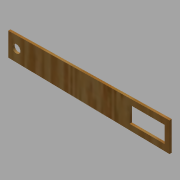
# Autodesk Inventor part: segment2b
Saved by Autodesk Inventor 2013 (Build 170138000, 138)
## iProperties
Created: 2014-10-09
Part Number: segment2b
Material: Plywood, Finish
Document SubType Name: Modeling
Designer: Masta
Density: 0.552 g/cm^3
Mass: 32.6528 g
Surface Area: 247.953 cm^2
Volume: 59.1536 cm^3
Author: Masta
Autodesk Inventor part; units mm, degrees
ref_plane "YZ Plane" through (0, 0, 0) normal (1, 0, 0) x (0, 1, 0)
ref_plane "XZ Plane" through (0, 0, 0) normal (0, 1, 0) x (-1, 0, 0)
ref_plane "XY Plane" through (0, 0, 0) normal (0, 0, 1) x (1, 0, 0)
sketch "Sketch2" plane through (0, 0, 0) normal (0, 1, 0) x (-1, 0, 0)
  circle A0 centre (188.3525, 14.1838) radius 2 projected
  circle A1 centre (143.3599, 14.996) radius 2 projected
  circle A2 centre (98.3672, 15.8081) radius 2 projected
  circle A3 centre (53.3745, 16.6203) radius 2 projected
  circle A4 centre (62, 0) radius 2.25 projected
  circle A5 centre (199, 0) radius 2.25 projected
  circle A6 centre (214.5, 0) radius 1.5 projected
  line L0 (217, 7) -> (217, -7) projected
  line L1 (217, 7) -> (247, 7) projected
  line L2 (247, 7) -> (247, -7) projected
  line L3 (217, -7) -> (247, -7) projected
  circle A7 centre (249.5, 0) radius 1.5 projected
  line L4 (254, 20) -> (254, -20) projected
  line L5 (254, 20) -> (-23, 25) projected
  line L6 (-23, 25) -> (-23, -25) projected
  line L7 (254, -20) -> (-23, -25) projected
  circle A8 centre (50, -8.5) radius 1.5 projected
  circle A9 centre (-19, -8.5) radius 1.5 projected
  line L8 (45.5, 14.25) -> (45.5, -14.25) projected
  line L9 (-14.5, -14.25) -> (45.5, -14.25) projected
  line L10 (-14.5, 14.25) -> (-14.5, -14.25) projected
  line L11 (-14.5, 14.25) -> (45.5, 14.25) projected
  circle A10 centre (-19, 8.5) radius 1.5 projected
  circle A11 centre (50, 8.5) radius 1.5 projected
  circle A12 centre (240, 0) radius 1.2295 construction
  circle A13 centre (240, 0) radius 7
  point P0 (0, 0)
  dimension "d77" = 14
  dimension "d28" = 18.5
  dimension "d37" = 20
  dimension "d38" = 20
  dimension "d39" = 42
  dimension "d40" = 21
  dimension "d41" = 50
  dimension "d42" = 10
  dimension "d43" = 10.5
  dimension "d52" = 240
  dimension "d53" = 14
  dimension "d54" = 9.5
  dimension "d62" = 10
  dimension "d73" = 274
  dimension "d74" = 20
  constraints: 1 centre point, 1 coincident
  measures "d77" diameter of A13
extrude "Extrusion2" add sketch "Sketch2" along normal blind 4 contours A0 | A1 | A2 | A3 | A6 | L1 A13 L3 L0 | L1 L2 A13 | A13 L2 L3 | A7 | L4 L7 L6 L5 | A8 | A9 | A10 | A11
body "Solid1"
body "Solid2"
